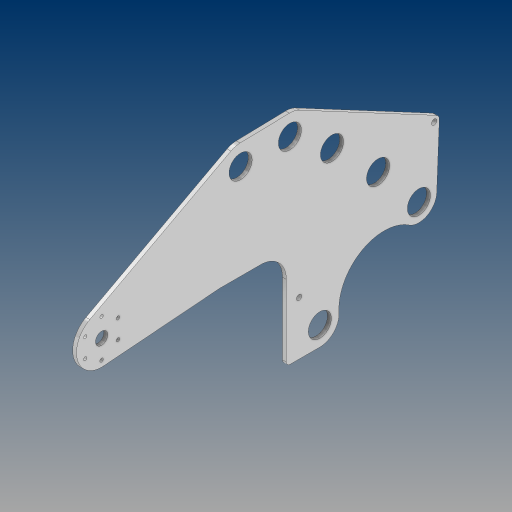
# Autodesk Inventor part: Intake Roller Plate
Saved by Autodesk Inventor 2024.3 (Build 283343000, 343)
## iProperties
Created: 2024-07-25
Part Number: Intake Roller Plate
Material: Aluminum 6061
Document SubType Name: Modeling
Designer: Kenji
Density: 2.7 g/cm^3
Appearance: Aluminum - Dark
Author: Kenji
Autodesk Inventor part; units mm, degrees
ref_plane "YZ Plane" through (0, 0, 0) normal (1, 0, 0) x (0, 1, 0)
ref_plane "XZ Plane" through (0, 0, 0) normal (0, 1, 0) x (-1, 0, 0)
ref_plane "XY Plane" through (0, 0, 0) normal (0, 0, 1) x (1, 0, 0)
sketch "Sketch1" plane through (0, 0, 0) normal (1, 0, 0) x (0, 1, 0)
  line L0 (127, 0) -> (127, -31.75) construction
  line L1 (95.25, -63.5) -> (31.75, -63.5) construction
  line L2 (0, -31.75) -> (0, 0) construction
  arc A0 (95.25, -63.5) -> (127, -31.75) centre (95.25, -31.75) ccw construction
  arc A1 (0, -31.75) -> (31.75, -63.5) centre (31.75, -31.75) ccw construction
  line L3 (0, 0) -> (0, 19.05) construction
  line L4 (0, 19.05) -> (-12.7, 19.05) construction
  line L5 (82.55, 19.05) -> (82.55, 292.1) construction
  circle A2 centre (82.55, 292.1) radius 25.4 construction
  circle A3 centre (82.55, 292.1) radius 31.75 construction
  circle A4 centre (231.775, 292.1) radius 25.4 construction
  circle A5 centre (231.775, 292.1) radius 31.75 construction
  line L6 (-12.7, 19.05) -> (82.55, 19.05) construction
  line L7 (127, 0) -> (0, 0) construction
  line L8 (-12.7, 19.05) -> (-12.7, -285.75) construction
  circle A6 centre (38.1, -178.6104) radius 50.8 construction
  circle A7 centre (96.0971, -228.0348) radius 25.4 construction
  circle A8 centre (96.0971, -228.0348) radius 14.2875
  circle A9 centre (153.6466, -177.3604) radius 25.4 construction
  circle A10 centre (153.6466, -177.3604) radius 14.2875
  circle A11 centre (246.5691, -67.8857) radius 22.225 construction
  circle A12 centre (246.5691, -67.8857) radius 25.4 construction
  circle A13 centre (246.5691, -67.8857) radius 14.2875
  line L9 (82.55, 19.05) -> (127, 19.05) construction
  line L10 (127, 19.05) -> (127, 0) construction
  circle A14 centre (153.6466, -177.3604) radius 22.225 construction
  circle A15 centre (96.0971, -228.0348) radius 22.225 construction
  circle A16 centre (25.4, -105.0867) radius 25.4 construction
  circle A17 centre (25.4, -105.0867) radius 23.8125 construction
  line L11 (25.4, -79.6867) -> (25.4, -63.5) construction
  circle A18 centre (207.8827, -120.1645) radius 25.4 construction
  circle A19 centre (207.8827, -120.1645) radius 22.225 construction
  circle A20 centre (207.8827, -120.1645) radius 14.2875
  line L12 (0, -105.0867) -> (-12.7, -105.0867) construction
  circle A21 centre (67.9471, -79.375) radius 6.477 construction
  circle A22 centre (25.4, -105.0867) radius 14.2875
  circle A23 centre (67.9471, -79.375) radius 3.2512
  circle A24 centre (84.9265, -152.658) radius 50.8 construction
  circle A25 centre (136.8978, -103.0238) radius 50.8 construction
  circle A26 centre (107.7568, -120.5556) radius 50.8 construction
  circle A27 centre (175.4762, -51.1988) radius 50.8 construction
  circle A28 centre (172.6204, -247.0086) radius 3.2512
  circle A29 centre (245.0871, -6.69) radius 14.2875
  circle A30 centre (245.0871, -6.69) radius 22.225 construction
  line L13 (178.2916, -250.0306) -> (268.9852, -79.8305)
  line L14 (207.8827, -120.1645) -> (153.6466, -177.3604) construction
  line L15 (153.6466, -177.3604) -> (96.0971, -228.0348) construction
  line L16 (82.55, 19.05) -> (31.75, 19.05) construction
  line L17 (31.75, 19.05) -> (31.75, 292.1) construction
  line L18 (31.75, 292.1) -> (82.55, 292.1) construction
  arc A31 (268.9852, -79.8305) -> (271.9617, -67.2708) centre (246.5691, -67.8857) ccw
  circle A32 centre (177.8, 21.6842) radius 50.8 construction
  circle A33 centre (245.0871, -6.69) radius 7.62 construction
  line L19 (-12.7, -285.75) -> (571.5, -285.75) construction
  line L20 (571.5, -285.75) -> (571.5, 292.1) construction
  line L21 (31.75, 292.1) -> (571.5, 292.1) construction
  line L22 (127, 19.05) -> (571.5, 19.05) construction
  circle A34 centre (146.5717, 165.8007) radius 7.62
  circle A35 centre (146.5717, 165.8007) radius 23.495 construction
  circle A36 centre (170.0667, 165.8007) radius 2.0828
  circle A37 centre (146.5717, 165.8007) radius 27.94 construction
  line L23 (115.5542, 163.3402) -> (126.985, 19.2385)
  circle A38 centre (146.5717, 165.8007) radius 31.115 construction
  arc A39 (174.0233, 180.4483) -> (115.5542, 163.3402) centre (146.5717, 165.8007) ccw
  circle A40 centre (158.3192, 186.1479) radius 2.0828
  circle A41 centre (134.8242, 186.1479) radius 2.0828
  circle A42 centre (123.0767, 165.8007) radius 2.0828
  circle A43 centre (134.8242, 145.4534) radius 2.0828
  circle A44 centre (158.3192, 145.4534) radius 2.0828
  line L24 (-12.7, -63.5) -> (368.3, -63.5) construction
  arc A45 (77.5036, -215.8597) -> (95.1813, -250.2409) centre (96.0971, -228.0348) ccw
  circle A46 centre (172.6204, -247.0086) radius 6.4262 construction
  line L25 (172.6204, -253.4348) -> (95.1813, -250.2409)
  arc A47 (172.6204, -253.4348) -> (178.2916, -250.0306) centre (172.6204, -247.0086) ccw
  line L26 (368.3, -63.5) -> (368.3, -285.75) construction
  line L27 (7.043, -120.2542) -> (81.9407, -210.9016) construction
  circle A48 centre (67.9471, -79.375) radius 6.35 construction
  line L28 (127, 18.8609) -> (127, -31.75)
  line L29 (95.25, -63.5) -> (6.3627, -63.5)
  line L30 (1.5875, -68.2752) -> (1.5875, -105.0867)
  arc A49 (6.3627, -63.5) -> (1.5875, -68.2752) centre (6.3627, -68.2752) ccw
  arc A50 (95.25, -63.5) -> (127, -31.75) centre (95.25, -31.75) ccw
  arc A51 (127, 18.8609) -> (126.985, 19.2385) centre (122.2248, 18.8609) ccw
  arc A52 (1.5875, -105.0867) -> (26.8912, -128.8524) centre (25.4, -105.0867) ccw
  circle A53 centre (245.0871, -6.69) radius 25.4 construction
  arc A54 (77.5036, -215.8597) -> (26.8912, -128.8524) centre (30.4159, -185.0264) ccw
  line L31 (245.0871, -6.69) -> (246.5691, -67.8857) construction
  line L32 (271.9617, -67.2708) -> (270.4797, -6.0751)
  circle A55 centre (177.8, -35.0642) radius 50.8 construction
  line L33 (174.0233, 180.4483) -> (267.4966, 5.2672)
  arc A56 (270.4797, -6.0751) -> (267.4966, 5.2672) centre (245.0871, -6.69) ccw
  point P0 (-12.7, -178.6104)
  point P1 (179.0466, -177.3604)
  point P2 (104.775, 19.05)
  point P3 (179.0466, -247.0086)
  point P4 (96.0971, -253.4348)
  point P5 (127, -63.5)
  point P6 (1.5875, -63.5)
  dimension "d58" = 101.6
  dimension "d284" = 46.99
  dimension "d388" = 50.8
  dimension "d2" = 31.75
  dimension "d3" = 19.05
  dimension "d4" = 12.7
  dimension "d7" = 273.05
  dimension "d8" = 50.8
  dimension "d9" = 6.35
  dimension "d10" = 50.8
  dimension "d11" = 6.35
  dimension "d12" = 149.225
  dimension "d14" = 127
  dimension "d16" = 304.8
  dimension "d175" = 31.75
  dimension "d180" = 50.8
  dimension "d181" = 1.5875
  dimension "d187" = 31.75
  dimension "d189" = 12.7
  dimension "d191" = 12.954
  dimension "d192" = 28.575
  dimension "d201" = 6.5024
  dimension "d207" = 101.6
  dimension "d208" = 101.6
  dimension "d210" = 130.175
  dimension "d214" = 15.875
  dimension "d216" = 101.6
  dimension "d218" = 6.5024
  dimension "d220" = 143.1895
  dimension "d221" = 155.574
  dimension "d236" = 50.8
  dimension "d237" = 44.45
  dimension "d267" = 15.24
  dimension "d271" = 584.2
  dimension "d283" = 15.24
  dimension "d285" = 4.1656
  dimension "d290" = 55.88
  dimension "d292" = 3.175
  dimension "d313" = 146.7507
  dimension "d318" = 114.8217
  dimension "d321" = 360
  dimension "d323" = 381
  dimension "d328" = 3.175
  dimension "d336" = 12.7
  dimension "d339" = 4.7752
  dimension "d340" = 31.75
  dimension "d341" = 4.7752
  dimension "d343" = 33.0042
  dimension "d344" = 64.0217
  dimension "d361" = 61.2137
  dimension "d375" = 16.1867
  dimension "d376" = 108.7971
  dimension "d377" = 76.6801
  dimension "d379" = 101.6
  dimension "d389" = 3.175
  dimension "d394" = 56.2845
  dimension "d395" = 44.45
  constraints: 69 end point, 52 centre point, 39 point on circle, 33 tangent, 20 point on line, 13 coincident, 13 equal radius, 11 perpendicular, 9 horizontal alignment, 8 concentric, 4 horizontal, 4 vertical, 4 vertical alignment, 3 parallel, 1 collinear, 1 midpoint, 34 other
  measures "d2" radius of A0
  measures "d3" distance of L2.end L3.end
  measures "d4" distance of L3.end L4.end
  measures "d7" distance of L5.start L5.end
  measures "d8" diameter of A2
  measures "d9" radial gap between concentric circles of A2 A3
  measures "d10" diameter of A4
  measures "d11" radial gap between concentric circles of A4 A5
  measures "d12" distance of L18.end A4.centre
  measures "d14" distance of L0.start L2.end
  measures "d16" distance of L4.end L8.end
  measures "d175" radius of A1
  measures "d180" diameter of A16
  measures "d181" radial gap between concentric circles of A16 A17
  measures "d187" distance of L0.start L0.end
  measures "d189" distance of L12.start L12.end
  measures "d191" diameter of A21
  measures "d192" diameter of A22
  measures "d201" diameter of A23
  measures "d207" diameter of A24
  measures "d208" diameter of A25
  measures "d210" distance of A21.centre A14.centre
  measures "d214" distance from line of L1 A21.centre
  measures "d216" diameter of A27
  measures "d218" diameter of A28
  measures "d220" distance of A0.centre A18.centre
  measures "d221" distance of A0.centre A11.centre
  measures "d236" distance of L5.start L16.end
  measures "d237" distance of L4.end L16.end
  measures "d267" diameter of A33
  measures "d271" distance of L8.end L19.end
  measures "d283" diameter of A34
  measures "d285" diameter of A36
  measures "d290" diameter of A37
  measures "d313" distance from line of L9 point (146.572, 165.801)
  measures "d318" distance from line of L17 point (146.572, 165.801)
  measures "d323" distance of L24.start L24.end
  measures "d328" radial gap between concentric circles of A28 A46
  measures "d336" diameter of A48
  measures "d339" radius of A49
  measures "d340" radius of A50
  measures "d341" radius of A51
  measures "d343" distance from line of L5 L23.start
  measures "d344" distance from line of L5 A37.centre
  measures "d361" distance of A30.centre A11.centre
  measures "d375" distance of L11.start L11.end
  measures "d376" distance from line of L8 A15.centre
  measures "d377" distance of L14.end L15.end
  measures "d379" diameter of A55
  measures "d394" radius of A54
  measures "d395" diameter of A15
extrude "Extrusion8" add sketch "Sketch1" along normal blind 4.7625
body "Solid7"
